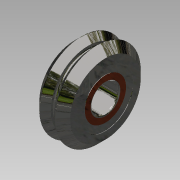
# Autodesk Inventor part: W2X
Saved by Autodesk Inventor 2020.1 (Build 241239000, 239)
## iProperties
Created: 2019-11-28
Part Number: W2X
Material: Generic
Catalog Web Link: https://www.bwc.com/dualvee.html
Description: Original DualVee Wheels-Original DualVee Wheels
Vendor: Bishop Wisecarver
Document SubType Name: Modeling
Designer: Autodesk Inc.
Manufacturer: BWC
Mass: 39 g
Surface Area: 27.8691 cm^2
Volume: 5.98954 cm^3
Density: 1 g/cm^3
Appearance: PSOLRGB-175-175-175
Category: FIRSTChoice
Company: Autodesk Inc.
PSOL_IDENT_0: {$CADENAS_DATA\23d-libs\bwc\dual_vee\wheels\original_dualvee_wheels.prj},163 {VTYP=3D},{NB=W2X},{LIN
PSOL_IDENT_1: A=W2X},{NN=Original DualVee Wheels},{DATE=01.07.2019 05:07:11},{GEOMDATE=12.02.2019 13:07:27},{VERSI
PSOL_IDENT_2: ON=},{LINEID=30},{WBVAR=},{WBNUMERIC=}  {NB=W2X},{LINA=W2X},{KT=DUMMY},{PN=W2X},{WS=WX Steel Seal/Sh
PSOL_IDENT_3: ield},{WSPN=X},{WSALG= 'X','WX Seal/Shield Steel', 'SSX','WSSX Seal/Shield Stainless Steel','SS227',
PSOL_IDENT_4: 'WSS227 Shield Stainless Steel Krytox GPL227 Lubricant','SS300', 'WSS300 Stainless Steel Isoflex PD
PSOL_IDENT_5: L 300 (grease, no shields or seals)','SSCVAC', 'Wacuum Wheels Stainless Steel, Ceramic Balls (no shi
PSOL_IDENT_6: eld, no grease)','SSVAC', 'Wacuum Wheels Shielded Stainless Steel (vacuum grease GL 057)','DW2SSX', '
PSOL_IDENT_7: Washdown Sealed Wheels' },{SIZE=2},{D=1.210},{W=0.438},{B=0.3750},{VRI=0.500},{VRO=0.719},{WEIGHT=39
PSOL_IDENT_8: .0},{C=0.584},{R=0.028},{R1=0.024},{E=0.009},{RLN=2650},{RLLBF=596},{ALN=625},{ALLBF=141},{ORMAT=521
PSOL_IDENT_9: 00 Steel},{IRMAT=52100 Steel},{BMAT=52100 Steel},{RMAT=Nylon 6,6},{SHMAT=304 Stainless steel},{SMAT=
PSOL_IDENT_10: NBR+304 Stainless steel},{GREASE=Kluberplex BEM 34-132},{CFGFILTER=PN,WS,SIZE,D,W,B,VRI,VRO,WEIGHT,R
PSOL_IDENT_11: LN,RLLBF,ALN,ALLBF,ORMAT,IRMAT,BMAT,RMAT,SHMAT,SMAT,GREASE},{CATEGALG=Original Guide Wheel, Size 2,
PSOL_IDENT_12: Carbon Steel, Sealed/Shielded},{FEATALG=<li style=\" margin-top:0px; margin-bottom:0px; margin-left:
PSOL_IDENT_13: 0px; margin-right:0px; -qt-block-indent:0; text-indent:0px;\"><span style=\" font-size:11pt; font-we
PSOL_IDENT_14: ight:600;\">General purpose AISI 52100 carbon steel</span></li><li style=\" font-size:11pt; font-wei
PSOL_IDENT_15: ght:600;\" style=\" margin-top:0px; margin-bottom:0px; margin-left:0px; margin-right:0px; -qt-block-
PSOL_IDENT_16: indent:0; text-indent:0px;\">Double row angular contact ball bearing</li><li style=\" font-size:11pt
PSOL_IDENT_17: ; font-weight:600;\" style=\" margin-top:0px; margin-bottom:0px; margin-left:0px; margin-right:0px;
PSOL_IDENT_18: -qt-block-indent:0; text-indent:0px;\">Precision ground 90° vee inside or outside running surfaces</
PSOL_IDENT_19: li><li style=\" font-size:11pt; font-weight:600;\" style=\" margin-top:0px; margin-bottom:0px; margi
PSOL_IDENT_20: n-left:0px; margin-right:0px; -qt-block-indent:0; text-indent:0px;\">Hardened for heavy loads and du
PSOL_IDENT_21: rability</li><li style=\" font-size:11pt; font-weight:600;\" style=\" margin-top:0px; margin-bottom:
PSOL_IDENT_22: 0px; margin-left:0px; margin-right:0px; -qt-block-indent:0; text-indent:0px;\">Seal/Shield combinati
PSOL_IDENT_23: on to protect against contamination</li>},{DESCRALG=<span style=\" font-size:11pt; font-weight:600;\
PSOL_IDENT_24: ">DualVee WX series guide wheels are linear guide bearings with double row angular contact ball arra
PSOL_IDENT_25: ngement.   Precision ground 90° vee inside or outside surfaces can be employed to support loads and
PSOL_IDENT_26: provide smooth and quiet motion. Use with DualVee guide track for linear motion. Hybrid seal/shield
PSOL_IDENT_27: design with rubber inner seal and metal outer shield protects against particle contamination of all
PSOL_IDENT_28: sizes. Through bore allows mounting on bushings or journals. Internally lubricated with general purp
PSOL_IDENT_29: ose grease.</span>},{RATINGSALG=<span style=\" font-size:11pt; font-weight:600; color:#000000;\">Tem
PSOL_IDENT_30: perature Range:</span><span style=\" font-size:11pt; color:#000000;\"> -22°F to +212°F</span></p><p
PSOL_IDENT_31: style=\" margin-top:0px; margin-bottom:0px; margin-left:0px; margin-right:0px; -qt-block-indent:0; t
PSOL_IDENT_32: ext-indent:0px;\"><span style=\" font-size:11pt; font-weight:600; color:#000000;\">RoHS Compliant</s
PSOL_IDENT_33: pan>},{MATCOLALG=ORMAT( title=\"$var. ($desc.)\", format=\"$value(SRC=VALDESC).\" ),IRMAT( title=\"$
PSOL_IDENT_34: var. ($desc.)\", format=\"$value(SRC=VALDESC).\" ),BMAT( title=\"$var. ($desc.)\", format=\"$value(S
PSOL_IDENT_35: RC=VALDESC).\" ),RMAT( title=\"$var. ($desc.)\", format=\"$value(SRC=VALDESC).\" ),SHMAT( title=\"$v
PSOL_IDENT_36: ar. ($desc.)\", format=\"$value(SRC=VALDESC).\" ),SMAT( title=\"$var. ($desc.)\", format=\"$value(SR
PSOL_IDENT_37: C=VALDESC).\" ),GREASE( title=\"$var. ($desc.)\", format=\"$value(SRC=VALDESC).\" )},{MATCOL1=ORMAT(
PSOL_IDENT_38: title=\"$var. ($desc.)\", format=\"$value(SRC=VALDESC).\" ),IRMAT( title=\"$var. ($desc.)\", format=
PSOL_IDENT_39: \"$value(SRC=VALDESC).\" ),BMAT( title=\"$var. ($desc.)\", format=\"$value(SRC=VALDESC).\" ),RMAT( t
PSOL_IDENT_40: itle=\"$var. ($desc.)\", format=\"$value(SRC=VALDESC).\" ),SHMAT( title=\"$var. ($desc.)\", format=\
PSOL_IDENT_41: "$value(SRC=VALDESC).\" ),SMAT( title=\"$var. ($desc.)\", format=\"$value(SRC=VALDESC).\" ),GREASE(
PSOL_IDENT_42: title=\"$var. ($desc.)\", format=\"$value(SRC=VALDESC).\" )}
NN: Original DualVee Wheels
NT: Original DualVee Wheels
NB: W2X
NBSYN: $PN.
LINA: W2X
PN: W2X
WS: WX Steel Seal/Shield
SIZE: 2
D: 1.21
W: 0.438
B: 0.375
VRI: 0.5
VRO: 0.719
WEIGHT: 39
RLN: 2650
RLLBF: 596
ALN: 625
ALLBF: 141
ORMAT: 52100 Steel
IRMAT: 52100 Steel
BMAT: 52100 Steel
RMAT: Nylon 6,6
SHMAT: 304 Stainless steel
SMAT: NBR+304 Stainless steel
GREASE: Kluberplex BEM 34-132
SUPPLIER: BWC
ARTICLENO: W2X
BOMINFO: W2X
CREATOR: CADENAS GmbH
Title: W2X
Author: Autodesk Inc.
Comments: Original DualVee Wheels
Autodesk Inventor part; units mm, degrees
sketch "Sketch_1" plane through (0, 0, 0) normal (0, 0, 1) x (1, 0, 0)
  line L0 (4.953, 0) -> (-4.953, 0)
  line L1 (-5.5626, 7.4168) -> (-5.5626, 5.3721)
  arc A0 (-5.5626, 5.3721) -> (-4.953, 4.7625) centre (-4.953, 5.3721) ccw
  line L2 (-4.953, 4.7625) -> (4.953, 4.7625)
  arc A1 (4.953, 4.7625) -> (5.5626, 5.3721) centre (4.953, 5.3721) ccw
  line L3 (5.5626, 5.3721) -> (5.5626, 7.4168)
  line L4 (5.5626, 7.4168) -> (5.4483, 7.4168)
  line L5 (5.4483, 7.4168) -> (5.4483, 7.3025)
  line L6 (5.4483, 7.3025) -> (5.334, 7.3025)
  line L7 (5.334, 7.3025) -> (5.334, 10.1727)
  line L8 (5.334, 10.1727) -> (5.4483, 10.1727)
  line L9 (5.4483, 10.1727) -> (5.4483, 10.0584)
  line L10 (5.4483, 10.0584) -> (5.5626, 10.0584)
  line L11 (5.5626, 10.0584) -> (5.5626, 12.7)
  line L12 (5.5626, 12.7) -> (2.8956, 15.367)
  line L13 (2.8956, 15.367) -> (2.667, 15.367)
  line L14 (2.667, 15.367) -> (0.7112, 13.4112)
  line L15 (0.7112, 13.4112) -> (0.7112, 12.7)
  arc A2 (-0.7112, 12.7) -> (0.7112, 12.7) centre (0, 12.7) ccw
  line L16 (-0.7112, 12.7) -> (-0.7112, 13.4112)
  line L17 (-0.7112, 13.4112) -> (-2.667, 15.367)
  line L18 (-2.667, 15.367) -> (-2.8956, 15.367)
  line L19 (-2.8956, 15.367) -> (-5.5626, 12.7)
  line L20 (-5.5626, 12.7) -> (-5.5626, 10.0584)
  line L21 (-5.5626, 10.0584) -> (-5.4483, 10.0584)
  line L22 (-5.4483, 10.0584) -> (-5.4483, 10.1727)
  line L23 (-5.4483, 10.1727) -> (-5.334, 10.1727)
  line L24 (-5.334, 10.1727) -> (-5.334, 7.3025)
  line L25 (-5.334, 7.3025) -> (-5.4483, 7.3025)
  line L26 (-5.4483, 7.3025) -> (-5.4483, 7.4168)
  line L27 (-5.4483, 7.4168) -> (-5.5626, 7.4168)
  constraints: 56 end point, 6 point on circle, 3 centre point
revolve "Revolution1" add sketch "Sketch_1" angle 360 about axis through (4.953, 0, 0) along (1, 0, 0)
ref_plane "b_XY" through (-4.953, 4.7625, 0) normal (0, 0, 1) x (1, 0, 0)
ref_plane "b_YZ" through (-4.953, 4.7625, 0) normal (1, 0, 0) x (0, 1, 0)
ref_plane "b_ZX" through (-4.953, 4.7625, 0) normal (0, 1, 0) x (0, 0, 1)
ref_plane "b1_XY" through (-4.953, -4.7625, 0) normal (0, 0, 1) x (1, 0, 0)
ref_plane "b1_YZ" through (-4.953, -4.7625, 0) normal (1, 0, 0) x (0, 1, 0)
ref_plane "b1_ZX" through (-4.953, -4.7625, 0) normal (0, 1, 0) x (0, 0, 1)
ref_plane "d_XY" through (-2.7813, 15.367, 0) normal (0, 0, 1) x (1, 0, 0)
ref_plane "d_YZ" through (-2.7813, 15.367, 0) normal (1, 0, 0) x (0, 1, 0)
ref_plane "d_ZX" through (-2.7813, 15.367, 0) normal (0, 1, 0) x (0, 0, 1)
ref_plane "d1_XY" through (-2.7813, -15.367, 0) normal (0, 0, 1) x (1, 0, 0)
ref_plane "d1_YZ" through (-2.7813, -15.367, 0) normal (1, 0, 0) x (0, 1, 0)
ref_plane "d1_ZX" through (-2.7813, -15.367, 0) normal (0, 1, 0) x (0, 0, 1)
ref_plane "vri_XY" through (0, 12.7, 0) normal (0, 0, 1) x (1, 0, 0)
ref_plane "vri_YZ" through (0, 12.7, 0) normal (1, 0, 0) x (0, 1, 0)
ref_plane "vri_ZX" through (0, 12.7, 0) normal (0, 1, 0) x (0, 0, 1)
ref_plane "vri1_XY" through (5.5626, 0, 0) normal (0, 0, 1) x (1, 0, 0)
ref_plane "vri1_YZ" through (5.5626, 0, 0) normal (1, 0, 0) x (0, 1, 0)
ref_plane "vri1_ZX" through (5.5626, 0, 0) normal (0, 1, 0) x (0, 0, 1)
ref_plane "w_XY" through (-5.5626, 12.7, 0) normal (0, 0, 1) x (1, 0, 0)
ref_plane "w_YZ" through (-5.5626, 12.7, 0) normal (1, 0, 0) x (0, 1, 0)
ref_plane "w_ZX" through (-5.5626, 12.7, 0) normal (0, 1, 0) x (0, 0, 1)
ref_plane "w1_XY" through (5.5626, 12.7, 0) normal (0, 0, 1) x (1, 0, 0)
ref_plane "w1_YZ" through (5.5626, 12.7, 0) normal (1, 0, 0) x (0, 1, 0)
ref_plane "w1_ZX" through (5.5626, 12.7, 0) normal (0, 1, 0) x (0, 0, 1)
ref_plane "wheel_XY" through (5.5626, 0, 0) normal (1, 0, 0) x (0, 0, -1)
ref_plane "wheel_YZ" through (5.5626, 0, 0) normal (0, 0, -1) x (0, 1, 0)
ref_plane "wheel_ZX" through (5.5626, 0, 0) normal (0, 1, 0) x (1, 0, 0)
ref_plane "wheel2_XY" through (-5.5626, 0, 0) normal (1, 0, 0) x (0, 0, -1)
ref_plane "wheel2_YZ" through (-5.5626, 0, 0) normal (0, 0, -1) x (0, 1, 0)
ref_plane "wheel2_ZX" through (-5.5626, 0, 0) normal (0, 1, 0) x (1, 0, 0)
body "Solid1"
